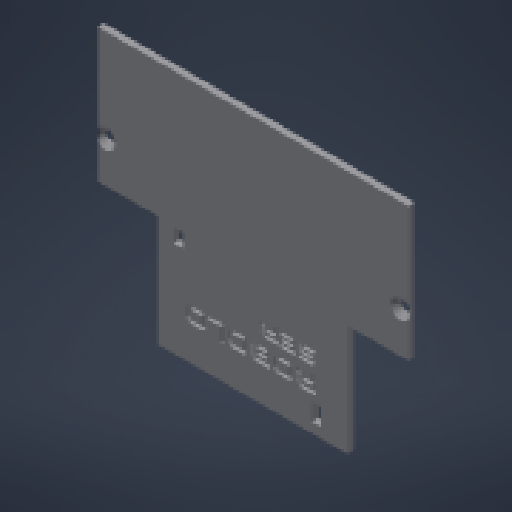
# Autodesk Inventor part: Dach_MocowaniePlytki
Saved by Autodesk Inventor 2023 (Build 270158000, 158)
## iProperties
Created: 2022-03-27
Part Number: Dach_MocowaniePlytki
Material: Ogólny
Document SubType Name: Modeling
Designer: Michał
Density: 1 g/cm^3
Appearance: Domyślna
Author: Michał
Autodesk Inventor part; units mm, degrees
ref_plane "YZ Plane" through (0, 0, 0) normal (1, 0, 0) x (0, 1, 0)
ref_plane "XZ Plane" through (0, 0, 0) normal (0, 1, 0) x (-1, 0, 0)
ref_plane "XY Plane" through (0, 0, 0) normal (0, 0, 1) x (1, 0, 0)
sketch "Szkic1" plane through (0, 0, 0) normal (0, 0, 1) x (1, 0, 0)
  line L0 (6.7, -3.9) -> (-52.8, -3.9)
  line L1 (-52.8, -3.9) -> (-52.8, -38.9)
  line L2 (-52.8, -38.9) -> (6.7, -38.9)
  line L3 (6.7, -38.9) -> (6.7, -3.9)
  line L4 (25.85, -3.9) -> (-72.15, -3.9)
  line L5 (-72.15, -3.9) -> (-72.15, 38.3115)
  line L6 (-72.15, 38.3115) -> (25.85, 38.3115)
  line L7 (25.85, 38.3115) -> (25.85, -3.9)
  line L8 (-1.5, -35.6277) -> (-4.5, -35.6277)
  line L9 (-4.5, -35.6277) -> (-4.5, -30.2332)
  line L10 (-4.5, -30.2332) -> (-1.5, -30.2332)
  line L11 (-1.5, -30.2332) -> (-1.5, -35.6277)
  line L12 (-45.2, -8.7637) -> (-48.2, -8.7637)
  line L13 (-48.2, -8.7637) -> (-48.2, -4.5195)
  line L14 (-48.2, -4.5195) -> (-45.2, -4.5195)
  line L15 (-45.2, -4.5195) -> (-45.2, -8.7637)
  line L16 (25.85, -39.1) -> (-72.15, -39.1) construction
  line L17 (25.85, 38.5115) -> (-72.15, 38.5115) construction
  line L18 (25.85, -3.9) -> (25.85, 38.5115) construction
  line L19 (-72.15, 38.7115) -> (-72.15, -3.9) construction
  line L20 (4.5, -35.6277) -> (-4.5, -35.6277) construction
  line L21 (-4.5, -30.2332) -> (4.5, -30.2332) construction
  line L22 (-45.2, -8.7637) -> (-50.8, -8.7637) construction
  line L23 (-45.8, -4.5195) -> (-45.2, -4.5195) construction
  line L24 (6.7, -4) -> (6.7, -34) projected
  line L25 (-52.8, -39.1) -> (-52.8, 10.9) construction
  point P0 (0, 0)
  point P1 (-4.8, -3.9)
  point P2 (-9.8, -3.9)
  dimension "d0" = 0.2
  dimension "d1" = 0.2
  dimension "d2" = 3
  dimension "d3" = 3
  constraints: 32 end point, 8 parallel, 4 horizontal, 4 perpendicular, 3 collinear, 2 point on line
  measures "d0" distance between parallel lines of L16 L2
  measures "d1" distance between parallel lines of L17 L6
  measures "d2" distance between parallel lines of L9 L11
  measures "d3" distance between parallel lines of L15 L13
extrude "Extrusion6" add sketch "Szkic1" along normal blind 2
sketch "Szkic2" plane through (0, 0, 2) normal (0, 0, 1) x (1, 0, 0)
  line L0 (-3.3, -28.9) -> (-14.5684, -28.9) construction
  line L1 (-14.5684, -28.9) -> (-14.5684, -24.3018) construction
  line L2 (-14.5684, -24.3018) -> (-3.3, -24.3018) construction
  line L3 (-3.3, -24.3018) -> (-3.3, -28.9) construction
  line L4 (-3.3, -20.3018) -> (-21.439, -20.3018) construction
  line L5 (-21.439, -20.3018) -> (-21.439, -15.3018) construction
  line L6 (-21.439, -15.3018) -> (-3.3, -15.3018) construction
  line L7 (-3.3, -15.3018) -> (-3.3, -20.3018) construction
  line L8 (-52.8, -38.9) -> (6.7, -38.9) construction
  line L9 (6.7, -38.9) -> (6.7, -3.9) construction
  line L10 (-9.6005, -23.0885) -> (-8.1066, -23.0885)
  line L11 (-8.1066, -23.0885) -> (-8.1066, -24.2997)
  line L12 (-8.1066, -24.2997) -> (-7.6519, -24.743)
  line L13 (-7.6519, -24.743) -> (-4.7978, -24.743)
  line L14 (-4.7978, -24.743) -> (-4.7978, -23.0885)
  line L15 (-4.7978, -23.0885) -> (-3.3038, -22.2327)
  line L16 (-3.3038, -22.2327) -> (-3.3038, -28.0327)
  line L17 (-3.3038, -28.0327) -> (-8.4734, -28.0327)
  line L18 (-8.4734, -28.0327) -> (-9.6005, -26.5158)
  line L19 (-9.6005, -26.5158) -> (-8.7447, -25.3657)
  line L20 (-8.7447, -25.3657) -> (-9.6005, -24.5061)
  line L21 (-9.6005, -24.5061) -> (-9.6005, -23.0885)
  line L22 (-8.0646, -26.4126) -> (-7.6672, -26.9323)
  line L23 (-7.6672, -26.9323) -> (-4.7978, -26.9323)
  line L24 (-4.7978, -26.9323) -> (-4.7978, -25.8663)
  line L25 (-4.7978, -25.8663) -> (-7.6634, -25.8663)
  line L26 (-7.6634, -25.8663) -> (-8.0646, -26.4126)
  line L27 (-16.8219, -24.2119) -> (-15.6986, -23.0885)
  line L28 (-15.6986, -23.0885) -> (-11.5721, -23.0885)
  line L29 (-11.5721, -23.0885) -> (-10.4487, -24.2119)
  line L30 (-10.4487, -24.2119) -> (-10.4487, -26.9094)
  line L31 (-10.4487, -26.9094) -> (-11.5721, -28.0327)
  line L32 (-11.5721, -28.0327) -> (-15.6986, -28.0327)
  line L33 (-15.6986, -28.0327) -> (-16.8219, -26.9094)
  line L34 (-16.8219, -26.9094) -> (-16.8219, -24.2119)
  line L35 (-15.3279, -24.1889) -> (-15.3279, -26.9323)
  line L36 (-15.3279, -26.9323) -> (-11.9427, -26.9323)
  line L37 (-11.9427, -26.9323) -> (-11.9427, -24.1889)
  line L38 (-11.9427, -24.1889) -> (-15.3279, -24.1889)
  line L39 (-23.9821, -24.6016) -> (-22.8588, -23.0809)
  line L40 (-22.8588, -23.0809) -> (-17.6204, -23.0809)
  line L41 (-17.6204, -23.0809) -> (-17.6204, -28.0327)
  line L42 (-17.6204, -28.0327) -> (-22.8588, -28.0327)
  line L43 (-22.8588, -28.0327) -> (-23.9821, -26.512)
  line L44 (-23.9821, -26.512) -> (-23.2791, -25.5568)
  line L45 (-23.2791, -25.5568) -> (-23.9821, -24.6016)
  line L46 (-22.3468, -24.6016) -> (-21.9838, -25.0524)
  line L47 (-21.9838, -25.0524) -> (-19.1144, -25.0524)
  line L48 (-19.1144, -25.0524) -> (-19.1144, -24.1889)
  line L49 (-19.1144, -24.1889) -> (-21.9838, -24.1889)
  line L50 (-21.9838, -24.1889) -> (-22.3468, -24.6016)
  line L51 (-22.3468, -26.512) -> (-21.9838, -26.9246)
  line L52 (-21.9838, -26.9246) -> (-19.1144, -26.9246)
  line L53 (-19.1144, -26.9246) -> (-19.1144, -26.0611)
  line L54 (-19.1144, -26.0611) -> (-21.9838, -26.0611)
  line L55 (-21.9838, -26.0611) -> (-22.3468, -26.512)
  line L56 (-31.1385, -24.2119) -> (-30.0152, -23.0885)
  line L57 (-30.0152, -23.0885) -> (-25.8887, -23.0885)
  line L58 (-25.8887, -23.0885) -> (-24.7653, -24.2119)
  line L59 (-24.7653, -24.2119) -> (-24.7653, -26.9094)
  line L60 (-24.7653, -26.9094) -> (-25.8887, -28.0327)
  line L61 (-25.8887, -28.0327) -> (-30.0152, -28.0327)
  line L62 (-30.0152, -28.0327) -> (-31.1385, -26.9094)
  line L63 (-31.1385, -26.9094) -> (-31.1385, -24.2119)
  line L64 (-29.6445, -24.1889) -> (-29.6445, -26.9323)
  line L65 (-29.6445, -26.9323) -> (-26.2593, -26.9323)
  line L66 (-26.2593, -26.9323) -> (-26.2593, -24.1889)
  line L67 (-26.2593, -24.1889) -> (-29.6445, -24.1889)
  line L68 (-37.6797, -24.1889) -> (-36.5717, -23.0809)
  line L69 (-36.5717, -23.0809) -> (-31.937, -23.0809)
  line L70 (-31.937, -23.0809) -> (-31.937, -28.0365)
  line L71 (-31.937, -28.0365) -> (-33.431, -28.9)
  line L72 (-33.431, -28.9) -> (-33.431, -24.1889)
  line L73 (-33.431, -24.1889) -> (-37.6797, -24.1889)
  line L74 (-44.2209, -24.2119) -> (-43.0976, -23.0885)
  line L75 (-43.0976, -23.0885) -> (-38.9711, -23.0885)
  line L76 (-38.9711, -23.0885) -> (-37.8478, -24.2119)
  line L77 (-37.8478, -24.2119) -> (-37.8478, -26.9094)
  line L78 (-37.8478, -26.9094) -> (-38.9711, -28.0327)
  line L79 (-38.9711, -28.0327) -> (-43.0976, -28.0327)
  line L80 (-43.0976, -28.0327) -> (-44.2209, -26.9094)
  line L81 (-44.2209, -26.9094) -> (-44.2209, -24.2119)
  line L82 (-42.727, -24.1889) -> (-42.727, -26.9323)
  line L83 (-42.727, -26.9323) -> (-39.3418, -26.9323)
  line L84 (-39.3418, -26.9323) -> (-39.3418, -24.1889)
  line L85 (-39.3418, -24.1889) -> (-42.727, -24.1889)
  line L86 (-9.2223, -17.3506) -> (-8.2539, -16.0397)
  line L87 (-8.2539, -16.0397) -> (-3.3033, -16.0397)
  line L88 (-3.3033, -16.0397) -> (-4.2519, -16.9883)
  line L89 (-4.2519, -16.9883) -> (-7.4996, -16.9883)
  line L90 (-7.4996, -16.9883) -> (-7.8026, -17.3506)
  line L91 (-7.8026, -17.3506) -> (-7.5029, -17.7327)
  line L92 (-7.5029, -17.7327) -> (-4.2453, -17.7327)
  line L93 (-4.2453, -17.7327) -> (-3.3033, -18.9909)
  line L94 (-3.3033, -18.9909) -> (-4.2717, -20.3018)
  line L95 (-4.2717, -20.3018) -> (-9.2223, -20.3018)
  line L96 (-9.2223, -20.3018) -> (-8.2671, -19.3532)
  line L97 (-8.2671, -19.3532) -> (-5.026, -19.3532)
  line L98 (-5.026, -19.3532) -> (-4.713, -18.9909)
  line L99 (-4.713, -18.9909) -> (-5.026, -18.6088)
  line L100 (-5.026, -18.6088) -> (-8.2835, -18.6088)
  line L101 (-8.2835, -18.6088) -> (-9.2223, -17.3506)
  line L102 (-14.8613, -20.3018) -> (-13.9126, -19.3466)
  line L103 (-13.9126, -19.3466) -> (-11.047, -19.3466)
  line L104 (-11.047, -19.3466) -> (-11.047, -18.6022)
  line L105 (-11.047, -18.6022) -> (-14.2387, -18.6022)
  line L106 (-14.2387, -18.6022) -> (-13.3692, -17.7327)
  line L107 (-13.3692, -17.7327) -> (-11.047, -17.7327)
  line L108 (-11.047, -17.7327) -> (-11.047, -16.9883)
  line L109 (-11.047, -16.9883) -> (-14.7097, -16.9883)
  line L110 (-14.7097, -16.9883) -> (-13.7545, -16.0331)
  line L111 (-13.7545, -16.0331) -> (-9.7592, -16.0331)
  line L112 (-9.7592, -16.0331) -> (-9.7592, -20.3018)
  line L113 (-9.7592, -20.3018) -> (-14.8613, -20.3018)
  line L114 (-20.7111, -16.0397) -> (-19.4232, -16.0397)
  line L115 (-19.4232, -16.0397) -> (-19.4232, -17.0838)
  line L116 (-19.4232, -17.0838) -> (-19.0312, -17.4659)
  line L117 (-19.0312, -17.4659) -> (-16.5708, -17.4659)
  line L118 (-16.5708, -17.4659) -> (-16.5708, -16.0397)
  line L119 (-16.5708, -16.0397) -> (-15.2829, -15.3018)
  line L120 (-15.2829, -15.3018) -> (-15.2829, -20.3018)
  line L121 (-15.2829, -20.3018) -> (-19.7394, -20.3018)
  line L122 (-19.7394, -20.3018) -> (-20.7111, -18.9942)
  line L123 (-20.7111, -18.9942) -> (-19.9733, -18.0028)
  line L124 (-19.9733, -18.0028) -> (-20.7111, -17.2617)
  line L125 (-20.7111, -17.2617) -> (-20.7111, -16.0397)
  line L126 (-19.387, -18.9053) -> (-19.0444, -19.3532)
  line L127 (-19.0444, -19.3532) -> (-16.5708, -19.3532)
  line L128 (-16.5708, -19.3532) -> (-16.5708, -18.4343)
  line L129 (-16.5708, -18.4343) -> (-19.0411, -18.4343)
  line L130 (-19.0411, -18.4343) -> (-19.387, -18.9053)
  point P0 (0, 0)
  dimension "d12" = 4.5982
  dimension "d14" = 18.139
  dimension "d15" = 5
  dimension "d48" = 4
  dimension "d51" = 10
  dimension "d52" = 10
  constraints: 1 collinear, 4 other
  measures "d12" distance between parallel lines of L0 L2
  measures "d14" distance of L4.start L4.end
  measures "d15" distance of L6.end L4.start
  measures "d48" distance between parallel lines of L2 L4
  measures "d51" distance between parallel lines of L8 L0
  measures "d52" distance between parallel lines of L9 L3
extrude "Wyciągnięcie proste2" cut sketch "Szkic2" against normal blind 1
sketch "Sketch8" plane through (0, 0, 2) normal (0, 0, 1) x (1, 0, 0)
  circle A0 centre (23.35, 9.1) radius 1.2295 construction
  circle A1 centre (-69.65, 9.1) radius 1.2295 construction
  point P0 (0, 0)
  constraints: 2 centre point, 2 coincident, 4 other
hole "Hole3" at (23.35, 9.1, 2) at (-69.65, 9.1, 2) direction (0, 0, -1) diameter 3.4 end through all countersink diameter 6.3 countersink angle 90 clearance for "Countersunk Flat Head Screw ISO 2009/7046" size "M3" standard "ISO"
sketch "Sketch9" plane through (0, 0, 2) normal (0, 0, 1) x (1, 0, 0)
  line L0 (-10.4487, -24.2119) -> (-10.4487, -26.9094) projected
  line L1 (-10.4487, -26.9094) -> (-11.5721, -28.0327) projected
  line L2 (-11.5721, -28.0327) -> (-15.6986, -28.0327) projected
  line L3 (-15.6986, -28.0327) -> (-16.8219, -26.9094) projected
  line L4 (-16.8219, -26.9094) -> (-16.8219, -24.2119) projected
  line L5 (-16.8219, -24.2119) -> (-15.6986, -23.0885) projected
  line L6 (-15.6986, -23.0885) -> (-11.5721, -23.0885) projected
  line L7 (-11.5721, -23.0885) -> (-10.4487, -24.2119) projected
  line L8 (-11.9427, -24.1889) -> (-15.3279, -24.1889) projected
  line L9 (-11.9427, -26.9323) -> (-11.9427, -24.1889) projected
  line L10 (-15.3279, -26.9323) -> (-11.9427, -26.9323) projected
  line L11 (-15.3279, -24.1889) -> (-15.3279, -26.9323) projected
  point P0 (0, 0)
extrude "Extrusion7" add sketch "Sketch9" along normal up to surface (1 mm away) from surface at -1
sketch "Sketch10" plane through (0, 0, 2) normal (0, 0, 1) x (1, 0, 0)
  circle A0 centre (-13.6105, -25.5568) radius 1.25
  line L0 (-15.0399, -23.0809) -> (-12.181, -23.0809)
  line L1 (-12.181, -23.0809) -> (-10.7516, -25.5568)
  line L2 (-10.7516, -25.5568) -> (-12.181, -28.0327)
  line L3 (-12.181, -28.0327) -> (-15.0399, -28.0327)
  line L4 (-15.0399, -28.0327) -> (-16.4694, -25.5568)
  line L5 (-16.4694, -25.5568) -> (-15.0399, -23.0809)
  line L6 (-10.7516, -25.5568) -> (-9.6005, -25.5568) construction
  line L7 (-9.6005, -24.5061) -> (-9.6005, -23.0885) construction
  line L8 (-3.3038, -28.0327) -> (-8.4734, -28.0327) construction
  line L9 (-22.8588, -23.0809) -> (-17.6204, -23.0809) construction
  line L10 (-16.4694, -25.5568) -> (-17.6204, -25.5568) construction
  line L11 (-17.6204, -23.0809) -> (-17.6204, -28.0327) construction
  point P0 (0, 0)
  dimension "d62" = 2.5
  constraints: 16 end point, 3 collinear, 3 horizontal, 1 centre point, 1 coincident, 1 midpoint, 1 point on line, 13 other
  measures "d62" diameter of A0
extrude "Extrusion8" cut sketch "Sketch10" along normal up to surface (1 mm away) from surface at -1
